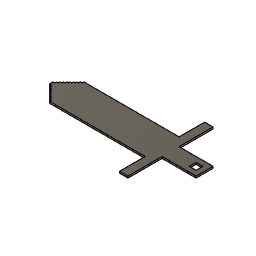
Pixel sword v1 (Autodesk Fusion 360 design; units mm, degrees)
Autodesk Fusion 360 part; units mm, degrees
sketch "Sketch1" plane through (0, 0, 0) normal (0, 0, 1) x (1, 0, 0)
  line L0 (45, 15) -> (30, 15)
  line L1 (30, 15) -> (30, 25)
  line L2 (30, 25) -> (45, 25)
  line L3 (30, 25) -> (30, 40)
  line L4 (30, 40) -> (30, 0)
  line L5 (25, 0) -> (25, 40)
  line L6 (25, 30) -> (-25, 30)
  line L7 (25, 10) -> (-25, 10)
  line L8 (-25, 10) -> (-30, 10)
  line L9 (-30, 30) -> (-25, 30)
  line L10 (-30, 30) -> (-31, 30)
  line L11 (-31, 30) -> (-31, 29)
  line L12 (-31, 29) -> (-32, 29)
  line L13 (-32, 29) -> (-32, 28)
  line L14 (-32, 28) -> (-33, 28)
  line L15 (-33, 28) -> (-33, 27)
  line L16 (-33, 27) -> (-34, 27)
  line L17 (-34, 27) -> (-34, 26)
  line L18 (-34, 26) -> (-35, 26)
  line L19 (-35, 26) -> (-35, 25)
  line L20 (-35, 25) -> (-36, 25)
  line L21 (-36, 25) -> (-36, 24)
  line L22 (-36, 24) -> (-37, 24)
  line L23 (-37, 24) -> (-37, 23)
  line L24 (-37, 23) -> (-38, 23)
  line L25 (-38, 23) -> (-38, 22)
  line L26 (-38, 22) -> (-39, 22)
  line L27 (-39, 22) -> (-39, 21)
  line L28 (-39, 21) -> (-40, 21)
  line L29 (-40, 21) -> (-40, 20)
  line L30 (-30, 10) -> (-31, 10)
  line L31 (-31, 10) -> (-31, 11)
  line L32 (-31, 11) -> (-32, 11)
  line L33 (-32, 11) -> (-32, 12)
  line L34 (-32, 12) -> (-33, 12)
  line L35 (-33, 12) -> (-33, 13)
  line L36 (-33, 13) -> (-34, 13)
  line L37 (-34, 13) -> (-34, 14)
  line L38 (-34, 14) -> (-35, 14)
  line L39 (-35, 14) -> (-35, 15)
  line L40 (-35, 15) -> (-36, 15)
  line L41 (-36, 15) -> (-36, 16)
  line L42 (-36, 16) -> (-37, 16)
  line L43 (-37, 16) -> (-37, 17)
  line L44 (-37, 17) -> (-38, 17)
  line L45 (-38, 17) -> (-38, 18)
  line L46 (-38, 18) -> (-39, 18)
  line L47 (-39, 18) -> (-39, 19)
  line L48 (-39, 19) -> (-40, 19)
  line L49 (-40, 19) -> (-40, 20)
  line L50 (-40, 20.5) -> (-41, 20.5)
  line L51 (-41, 20.5) -> (-41, 19.5)
  line L52 (-41, 19.5) -> (-40, 19.5)
  line L53 (-41, 20.2859) -> (-41.5, 20.2859)
  line L54 (-41.5, 20.2859) -> (-41.5, 19.8)
  line L55 (30, 0) -> (30, -5)
  line L56 (25, 0) -> (25, -5)
  line L57 (25, -5) -> (30, -5)
  line L58 (30, 40) -> (30, 45)
  line L59 (30, 45) -> (25, 45)
  line L60 (25, 45) -> (25, 40)
  line L61 (45, 25) -> (50, 25)
  line L62 (50, 25) -> (50, 15)
  line L63 (50, 15) -> (45, 15)
  line L64 (43, 22) -> (43, 18)
  line L65 (43, 18) -> (47, 18)
  line L66 (47, 18) -> (47, 22)
  line L67 (47, 22) -> (43, 22)
  constraint perpendicular L0 L1
  constraint perpendicular L2 L3
  constraint perpendicular L2 L4
  constraint coincident L5 L6.start
  constraint perpendicular L5 L6
  constraint coincident L5 L7.start
  constraint perpendicular L5 L7
  constraint perpendicular L5 L8
  constraint perpendicular L5 L9
  constraint perpendicular L10 L11
  constraint perpendicular L11 L12
  constraint perpendicular L12 L13
  constraint perpendicular L13 L14
  constraint perpendicular L14 L15
  constraint perpendicular L15 L16
  constraint perpendicular L16 L17
  constraint perpendicular L17 L18
  constraint perpendicular L18 L19
  constraint perpendicular L19 L20
  constraint perpendicular L20 L21
  constraint perpendicular L21 L22
  constraint perpendicular L22 L23
  constraint perpendicular L23 L24
  constraint perpendicular L24 L25
  constraint perpendicular L25 L26
  constraint perpendicular L26 L27
  constraint perpendicular L27 L28
  constraint perpendicular L30 L31
  constraint perpendicular L31 L32
  constraint perpendicular L32 L33
  constraint perpendicular L33 L34
  constraint perpendicular L34 L35
  constraint perpendicular L35 L36
  constraint perpendicular L36 L37
  constraint perpendicular L37 L38
  constraint perpendicular L38 L39
  constraint perpendicular L39 L40
  constraint perpendicular L40 L41
  constraint perpendicular L41 L42
  constraint perpendicular L42 L43
  constraint perpendicular L43 L44
  constraint perpendicular L44 L45
  constraint perpendicular L45 L46
  constraint perpendicular L46 L47
  constraint perpendicular L47 L48
  constraint midpoint L29 L50.start
  constraint perpendicular L29 L50
  constraint perpendicular L50 L51
  constraint midpoint L49 L52.end
  constraint coincident L51 L53.start
  constraint perpendicular L51 L53
  constraint perpendicular L48 L54
  constraint perpendicular L55 L57
  constraint perpendicular L58 L59
  constraint perpendicular L61 L62
  constraint perpendicular L61 L64
  constraint perpendicular L64 L65
  constraint perpendicular L65 L66
  constraint perpendicular L64 L67
extrude "Extrude1" add sketch "Sketch1" along normal blind 1 contours L0 L1 L2 L4 L61 L62 L63 | L1 L3 L4 L5 L55 L56 L57 L58 L59 L60 | L5 L6 L7 L8 L9 L10 L11 L12 L13 L14 L15 L16 L17 L18 L19 L20 L21 L22 L23 L24 L25 L26 L27 L28 L29 L30 L31 L32 L33 L34 L35 L36 L37 L38 L39 L40 L41 L42 L43 L44 L45 L46 L47 L48 L49
